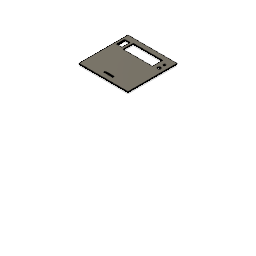
Lid (Autodesk Fusion 360 design; units mm, degrees)
Autodesk Fusion 360 part; units mm, degrees
sketch "Sketch1" plane through (0, 0, 0) normal (0, 1, 0) x (1, 0, 0)
  line L0 (0, 0) -> (120, 0)
  line L1 (120, 0) -> (120, -120)
  line L2 (120, -120) -> (0, -120)
  line L3 (0, -120) -> (0, 0)
  dimension "d11" = 120
  dimension "d12" = 120
  constraint horizontal L0
  constraint vertical L1
  constraint horizontal L2
  constraint vertical L3
  constraint coincident L0.start L3.end
  measures "d11" distance of L0.start L0.end
  measures "d12" distance of L0.end L1.end
extrude "Extrude1" add sketch "Sketch1" along normal blind 2.5
sketch "Sketch2" plane through (0, 0, 0) normal (0, -1, 0) x (1, 0, 0)
  line L0 (120, 120) -> (0, 120)
  line L1 (0, 120) -> (0, 0)
  line L2 (0, 0) -> (120, 0)
  line L3 (120, 0) -> (120, 120)
  line L4 (2.52, 117.48) -> (117.48, 117.48)
  line L5 (117.48, 117.48) -> (117.48, 2.52)
  line L6 (117.48, 2.52) -> (2.52, 2.52)
  line L7 (2.52, 2.52) -> (2.52, 117.48)
  line L8 (5.02, 114.98) -> (114.98, 114.98)
  line L9 (114.98, 114.98) -> (114.98, 5.02)
  line L10 (114.98, 5.02) -> (5.02, 5.02)
  line L11 (5.02, 5.02) -> (5.02, 114.98)
  line L12 (5.02, 114.98) -> (114.98, 5.02)
  line L13 (114.98, 114.98) -> (5.02, 5.02)
  line L14 (6.7878, 114.98) -> (114.98, 6.7878)
  line L15 (5.02, 113.2122) -> (113.2122, 5.02)
  line L16 (114.98, 113.2122) -> (6.7878, 5.02)
  line L17 (5.02, 6.7878) -> (113.2122, 114.98)
  dimension "d15" = 2.52
  dimension "d16" = 2.52
  dimension "d17" = 2.52
  dimension "d18" = 2.52
  dimension "d19" = 2.5
  dimension "d20" = 2.5
  dimension "d21" = 2.5
  dimension "d22" = 2.5
  dimension "d25" = 1.25
  dimension "d26" = 1.25
  dimension "d27" = 1.25
  dimension "d28" = 1.25
  constraint horizontal L4
  constraint vertical L5
  constraint horizontal L6
  constraint vertical L7
  constraint horizontal L8
  constraint vertical L9
  constraint horizontal L10
  constraint vertical L11
  constraint coincident L8 L14.start
  constraint coincident L9 L14.end
  constraint perpendicular L13 L14
  constraint coincident L11 L15.start
  constraint coincident L10 L15.end
  constraint parallel L14 L15
  constraint coincident L9 L16.start
  constraint coincident L10 L16.end
  constraint parallel L13 L16
  constraint coincident L11 L17.start
  constraint coincident L8 L17.end
  constraint perpendicular L14 L17
  measures "d15" distance of L1 L7
  measures "d16" distance of L0 L4
  measures "d17" distance of L3 L5
  measures "d18" distance of L2 L6
  measures "d19" distance of L5 L9
  measures "d20" distance of L4 L8
  measures "d21" distance of L6 L10
  measures "d22" distance of L7 L11
  measures "d25" distance of L12 L14
  measures "d26" distance of L12 L15
  measures "d27" distance of L13 L16
  measures "d28" distance of L13 L17
extrude "Extrude3" add sketch "Sketch2" along normal blind 3 contours L11 L12 L15 L17 | L8 L12 L14 L17 | L12 L13 L14 L17 | L12 L13 L15 L17 | L8 L13 L14 L17 | L11 L13 L15 L17 | L12 L13 L14 L16 | L12 L13 L15 L16 | L9 L13 L14 L16 | L10 L13 L15 L16 | L9 L12 L14 L16 | L10 L12 L15 L16
extrude "Extrude2" add sketch "Sketch2" along normal blind 3 contours L4 L5 L6 L7
move_body "Align1" bodies 1 to x (1, 0, 0) y (0, 1, 0) z (0, 0, 1) at (0, 50, 0)
sketch "Sketch3" plane through (0, 52.5, 0) normal (0, 1, 0) x (-1, 0, 0)
  line L0 (0, 120) -> (-120, 120)
  line L1 (-120, 120) -> (-120, 0)
  line L2 (-120, 0) -> (0, 0)
  line L3 (0, 0) -> (0, 120)
  line L4 (-24.5, 12) -> (-95.5, 12)
  line L5 (-95.5, 12) -> (-95.5, 36)
  line L6 (-95.5, 36) -> (-24.5, 36)
  line L7 (-24.5, 36) -> (-24.5, 12)
  line L8 (-49.25, 104.5) -> (-70.75, 104.5)
  line L9 (-70.75, 104.5) -> (-70.75, 108)
  line L10 (-70.75, 108) -> (-49.25, 108)
  line L11 (-49.25, 108) -> (-49.25, 104.5)
  line L12 (-5.8, 14) -> (-18.5, 14)
  line L13 (-18.5, 14) -> (-18.5, 33.05)
  line L14 (-18.5, 33.05) -> (-5.8, 33.05)
  line L15 (-5.8, 33.05) -> (-5.8, 14)
  circle A0 centre (-107.75, 19) radius 2.5
  circle A1 centre (-107.75, 32) radius 3.5
  dimension "d42" = 71
  dimension "d43" = 24
  dimension "d44" = 12
  dimension "d45" = 24.5
  dimension "d46" = 21.5
  dimension "d47" = 3.5
  dimension "d48" = 49.25
  dimension "d49" = 19.05
  dimension "d50" = 12.7
  dimension "d51" = 6
  dimension "d52" = 5
  dimension "d53" = 7
  dimension "d54" = 12.25
  dimension "d55" = 12.25
  dimension "d56" = 13
  dimension "d57" = 14
  dimension "d58" = 32
  dimension "d67" = 12
  constraint horizontal L4
  constraint vertical L5
  constraint horizontal L6
  constraint vertical L7
  constraint horizontal L8
  constraint vertical L9
  constraint horizontal L10
  constraint vertical L11
  constraint horizontal L12
  constraint vertical L13
  constraint horizontal L14
  constraint vertical L15
  measures "d42" distance of L4.start L4.end
  measures "d43" distance of L4.end L5.end
  measures "d44" distance of L2 L4
  measures "d45" distance of L1 L5
  measures "d46" distance of L8.start L8.end
  measures "d47" distance of L8.end L9.end
  measures "d48" distance of L1 L9
  measures "d49" distance of L12.start L14.end
  measures "d50" distance of L12.start L12.end
  measures "d51" distance of L7 L13
  measures "d52" diameter of A0
  measures "d53" diameter of A1
  measures "d54" distance of L1 A0.centre
  measures "d55" distance of L1 A1.centre
  measures "d56" distance of A0.centre A1.centre
  measures "d57" distance of L2 L12
  measures "d58" distance of L2 A1.centre
  measures "d67" distance of L0 L10
extrude "Extrude4" cut sketch "Sketch3" against normal blind 8 contours L4 L5 L6 L7 | L8 L9 L10 L11 | L12 L13 L14 L15 | A0 | A1
sketch "Sketch4" plane through (0, 0, 0) normal (0, 1, 0) x (1, 0, 0)
sketch "Sketch5" plane through (0, 0, 0) normal (0, 1, 0) x (1, 0, 0)
  line L0 (27.5994, -29.3672) -> (6.4946, -29.3672)
  line L1 (6.4946, -29.3672) -> (6.4946, -10.3939)
  line L2 (6.4946, -10.3939) -> (27.5994, -10.3939)
  line L3 (27.5994, -10.3939) -> (27.5994, -29.3672)
  constraint horizontal L0
  constraint vertical L1
  constraint horizontal L2
  constraint vertical L3
extrude "Extrude5" cut sketch "Sketch5" along normal blind 3 from surface at 47
sketch "Sketch6" plane through (0, 0, 0) normal (0, 1, 0) x (1, 0, 0)
  line L0 (30, -39) -> (99, -39)
  line L1 (99, -39) -> (99, -12)
  line L2 (99, -12) -> (30, -12)
  line L3 (30, -12) -> (30, -39)
  constraint horizontal L0
  constraint vertical L1
  constraint horizontal L2
  constraint vertical L3
extrude "Extrude6" cut sketch "Sketch6" along normal blind 3 from surface at 47
move_body "Align2" bodies 1 to x (1, 0, 0) y (0, 1, 0) z (0, 0, 1) at (-120, 0, 0)
move_body "Align3" bodies 1 to x (1, 0, 0) y (0, 1, 0) z (0, 0, 1) at (0, 0, 120)
move_body "Align4" bodies 1 to x (1, 0, 0) y (0, 1, 0) z (0, 0, 1) at (0, 0, -240)
move_body "Align5" bodies 1 to x (1, 0, 0) y (0, 1, 0) z (0, 0, 1) at (0, 0, 0)
sketch "Sketch7" plane through (0, 47, 0) normal (0, -1, 0) x (1, 0, 0)
  line L0 (-21, -97.2322) -> (-21, -100.7678)
  line L1 (-21, -100.7678) -> (-6.7878, -114.98)
  line L2 (-6.7878, -114.98) -> (-113.2122, -114.98)
  line L3 (-113.2122, -114.98) -> (-107.8383, -109.6061)
  line L4 (-107.8383, -109.6061) -> (-111.3739, -109.6061)
  line L5 (-111.3739, -109.6061) -> (-114.98, -113.2122)
  line L6 (-114.98, -113.2122) -> (-114.98, -6.7878)
  line L7 (-114.98, -6.7878) -> (-61.7678, -60)
  line L8 (-61.7678, -60) -> (-82.7678, -81)
  line L9 (-82.7678, -81) -> (-79.2322, -81)
  line L10 (-79.2322, -81) -> (-60, -61.7678)
  line L11 (-60, -61.7678) -> (-40.7678, -81)
  line L12 (-40.7678, -81) -> (-37.2322, -81)
  line L13 (-37.2322, -81) -> (-58.2322, -60)
  line L14 (-58.2322, -60) -> (-5.02, -6.7878)
  line L15 (-5.02, -6.7878) -> (-5.02, -113.2122)
  line L16 (-5.02, -113.2122) -> (-21, -97.2322)
  line L17 (-117.48, -117.48) -> (-2.52, -117.48)
  line L18 (-2.52, -117.48) -> (-2.52, -2.52)
  line L19 (-2.52, -2.52) -> (-117.48, -2.52)
  line L20 (-117.48, -2.52) -> (-117.48, -117.48)
  line L21 (-113.2122, -5.02) -> (-6.7878, -5.02)
  line L22 (-6.7878, -5.02) -> (-60, -58.2322)
  line L23 (-60, -58.2322) -> (-113.2122, -5.02)
  line L24 (-4.52, -117.48) -> (-2.52, -115.48)
  line L25 (-2.52, -115.48) -> (-2.52, -117.48)
  line L26 (-4.52, -117.48) -> (-2.52, -117.48)
  line L27 (-115.48, -117.48) -> (-117.48, -115.48)
  line L28 (-115.48, -117.48) -> (-117.48, -117.48)
  line L29 (-117.48, -117.48) -> (-117.48, -115.48)
  line L30 (-115.48, -2.52) -> (-117.48, -4.52)
  line L31 (-115.48, -2.52) -> (-117.48, -2.52)
  line L32 (-117.48, -2.52) -> (-117.48, -4.52)
  line L33 (-4.52, -2.52) -> (-2.52, -4.52)
  line L34 (-2.52, -4.52) -> (-2.52, -2.52)
  line L35 (-2.52, -2.52) -> (-4.52, -2.52)
  dimension "d68" = 45
  dimension "d69" = 2
  dimension "d70" = 45
  dimension "d71" = 2
  dimension "d72" = 45
  dimension "d73" = 2
  dimension "d74" = 45
  dimension "d75" = 2
  constraint coincident L17 L24.start
  constraint coincident L18 L24.end
  constraint coincident L17.end L18.start
  constraint coincident L17 L27.start
  constraint coincident L20 L27.end
  constraint coincident L17.start L20.end
  constraint coincident L19 L30.start
  constraint coincident L20 L30.end
  constraint coincident L19.end L20.start
  constraint coincident L19 L33.start
  constraint coincident L18 L33.end
  constraint coincident L18.end L19.start
  measures "d68" angle of L17 L24
  measures "d69" distance of L24.start L17.end
  measures "d70" angle of L17 L27
  measures "d71" distance of L27.start L17.start
  measures "d72" angle of L30 L31
  measures "d73" distance of L30.start L19.end
  measures "d74" angle of L33 L35
  measures "d75" distance of L33.start L18.end
extrude "Extrude7" cut sketch "Sketch7" against normal up to surface (3 mm away) contours L17 L20 L27 L28 L29 | L17 L18 L24 L25 L26 | L19 L20 L30 L31 L32 | L18 L19 L33 L34 L35
chamfer "Chamfer1" distance 0.5 angle 45 8 edges at (-60, 47, -117.48) (-117.48, 47, -60) (-116.48, 47, -116.48) (-3.52, 47, -116.48) (-2.52, 47, -60) (-3.52, 47, -3.52) (-60, 47, -2.52) (-116.48, 47, -3.52)
sketch "Sketch8" plane through (0, 50, 0) normal (0, -1, 0) x (1, 0, 0)
  line L0 (-24.5, -84) -> (-24.5, -108)
  line L1 (-24.5, -108) -> (-95.5, -108)
  line L2 (-95.5, -108) -> (-95.5, -84)
  line L3 (-95.5, -84) -> (-24.5, -84)
  circle A0 centre (-12.25, -88) radius 3.5
  circle A1 centre (-12.25, -101) radius 2.5
  line L4 (-21, -100.7678) -> (-21, -97.2322)
  line L5 (-21, -97.2322) -> (-5.02, -113.2122)
  line L6 (-5.02, -113.2122) -> (-5.02, -6.7878)
  line L7 (-5.02, -6.7878) -> (-58.2322, -60)
  line L8 (-58.2322, -60) -> (-37.2322, -81)
  line L9 (-37.2322, -81) -> (-40.7678, -81)
  line L10 (-40.7678, -81) -> (-60, -61.7678)
  line L11 (-60, -61.7678) -> (-79.2322, -81)
  line L12 (-79.2322, -81) -> (-82.7678, -81)
  line L13 (-82.7678, -81) -> (-61.7678, -60)
  line L14 (-61.7678, -60) -> (-114.98, -6.7878)
  line L15 (-114.98, -6.7878) -> (-114.98, -113.2122)
  line L16 (-114.98, -113.2122) -> (-111.3739, -109.6061)
  line L17 (-111.3739, -109.6061) -> (-107.8383, -109.6061)
  line L18 (-107.8383, -109.6061) -> (-113.2122, -114.98)
  line L19 (-113.2122, -114.98) -> (-6.7878, -114.98)
  line L20 (-6.7878, -114.98) -> (-21, -100.7678)
  line L21 (-101.5, -86.95) -> (-101.5, -106)
  line L22 (-101.5, -106) -> (-114.2, -106)
  line L23 (-114.2, -106) -> (-114.2, -86.95)
  line L24 (-114.2, -86.95) -> (-101.5, -86.95)
  circle A2 centre (-97.48, -69) radius 2.5
  circle A3 centre (-97.48, -19) radius 2.5
  circle A4 centre (-22.48, -69) radius 2.5
  circle A5 centre (-22.48, -19) radius 2.5
  line L25 (-120, 0) -> (-120, -120)
  circle A6 centre (-89.98, -64) radius 2.5
  circle A7 centre (-89.98, -24) radius 2.5
  circle A8 centre (-29.98, -64) radius 2.5
  circle A9 centre (-29.98, -24) radius 2.5
  line L26 (-114.98, -113.2122) -> (-114.98, -6.7878)
  circle A10 centre (-22.48, -69) radius 0.5
  circle A11 centre (-29.98, -64) radius 0.5
  circle A12 centre (-29.98, -24) radius 0.5
  circle A13 centre (-22.48, -19) radius 0.5
  circle A14 centre (-89.98, -24) radius 0.5
  circle A15 centre (-97.48, -19) radius 0.5
  circle A16 centre (-89.98, -64) radius 0.5
  circle A17 centre (-97.48, -69) radius 0.5
  dimension "d79" = 5
  dimension "d80" = 5
  dimension "d81" = 5
  dimension "d82" = 5
  dimension "d83" = 50
  dimension "d84" = 15
  dimension "d85" = 50
  dimension "d86" = 15
  dimension "d87" = 75
  dimension "d89" = 17.5
  dimension "d90" = 5
  dimension "d91" = 5
  dimension "d92" = 5
  dimension "d93" = 5
  dimension "d94" = 40
  dimension "d95" = 40
  dimension "d96" = 60
  dimension "d97" = 25
  dimension "d98" = 20
  dimension "d99" = 1
  dimension "d100" = 1
  dimension "d101" = 1
  dimension "d102" = 1
  dimension "d103" = 1
  dimension "d104" = 1
  dimension "d105" = 1
  dimension "d106" = 1
  constraint concentric A4 A10
  constraint concentric A8 A11
  constraint concentric A9 A12
  constraint concentric A5 A13
  constraint concentric A7 A14
  constraint concentric A3 A15
  constraint concentric A6 A16
  constraint concentric A2 A17
  measures "d79" diameter of A2
  measures "d80" diameter of A3
  measures "d81" diameter of A5
  measures "d82" diameter of A4
  measures "d83" distance of A2.centre A3.centre
  measures "d84" distance of L3 A2.centre
  measures "d85" distance of A4.centre A5.centre
  measures "d86" distance of L3 A4.centre
  measures "d87" distance of A2.centre A4.centre
  measures "d89" distance of L15 A2.centre
  measures "d90" diameter of A6
  measures "d91" diameter of A7
  measures "d92" diameter of A8
  measures "d93" diameter of A9
  measures "d94" distance of A6.centre A7.centre
  measures "d95" distance of A8.centre A9.centre
  measures "d96" distance of A6.centre A8.centre
  measures "d97" distance of A6.centre L26
  measures "d98" distance of L3 A6.centre
  measures "d99" diameter of A10
  measures "d100" diameter of A11
  measures "d101" diameter of A12
  measures "d102" diameter of A13
  measures "d103" diameter of A14
  measures "d104" diameter of A15
  measures "d105" diameter of A16
  measures "d106" diameter of A17
extrude "Extrude8" add sketch "Sketch8" along normal up to surface (3 mm away) contours A2 | A3 | A4 | A5 | A6 | A7 | A8 | A9
